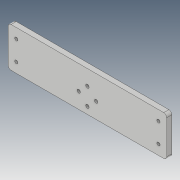
# Autodesk Inventor part: verticalAcrylicMount
Saved by Autodesk Inventor 2018 (Build 220112000, 112)
## iProperties
Created: 2020-02-23
Part Number: verticalAcrylicMount
Material: Generic
Document SubType Name: Modeling
Designer: anirudh
Density: 1 g/cm^3
Appearance: Default
Author: anirudh
Autodesk Inventor part; units mm, degrees
ref_plane "YZ Plane" through (0, 0, 0) normal (1, 0, 0) x (0, 1, 0)
ref_plane "XZ Plane" through (0, 0, 0) normal (0, 1, 0) x (-1, 0, 0)
ref_plane "XY Plane" through (0, 0, 0) normal (0, 0, 1) x (1, 0, 0)
sketch "Sketch1" plane through (0, 0, 0) normal (0, 0, 1) x (1, 0, 0)
  line L0 (0, 0) -> (149.225, 0)
  line L1 (149.225, 0) -> (149.225, -43.1292)
  line L2 (149.225, -43.1292) -> (0, -43.1292)
  line L3 (0, -43.1292) -> (0, 0)
  circle A0 centre (65.1125, -26.01) radius 1.85
  circle A1 centre (65.1125, -26.01) radius 1.85
  circle A2 centre (74.6125, -35.51) radius 1.85
  circle A3 centre (74.6125, -35.51) radius 1.85
  circle A4 centre (84.1125, -26.01) radius 1.85
  circle A5 centre (84.1125, -26.01) radius 1.85
  circle A6 centre (74.6125, -16.51) radius 1.85
  circle A7 centre (74.6125, -16.51) radius 1.85
  line L4 (0, 0) -> (8.89, 0)
  line L5 (149.225, 0) -> (140.335, 0)
  circle A8 centre (8.89, -10.7823) radius 1.75
  circle A9 centre (8.89, -32.3469) radius 1.75
  circle A10 centre (140.335, -10.7823) radius 1.75
  circle A11 centre (140.335, -32.3469) radius 1.75
  dimension "d0" = 149.225
  dimension "d1" = 43.1292
  dimension "d3" = 8.89
  dimension "d4" = 8.89
  dimension "d5" = 3.5
  dimension "d6" = 3.5
  dimension "d7" = 3.5
  dimension "d8" = 3.5
  constraints: 12 centre point, 12 end point, 4 coincident, 2 parallel, 2 point on line, 1 horizontal, 1 perpendicular
  measures "d0" distance of L1.end L2.end
  measures "d1" distance of L0.end L1.end
  measures "d3" distance of L0.start L4.end
  measures "d4" distance of L0.end L5.end
  measures "d5" diameter of A8
  measures "d6" diameter of A9
  measures "d7" diameter of A10
  measures "d8" diameter of A11
extrude "Extrusion1" add sketch "Sketch1" along normal blind 5.588
sketch "Sketch2" plane through (0, 0, 5.588) normal (0, 0, 1) x (1, 0, 0)
  line L0 (149.225, 0) -> (0, 0) projected
  line L1 (0, 0) -> (-11.4173, 0)
  line L2 (-11.4173, 0) -> (-11.4173, -43.1292)
  line L3 (-11.4173, -43.1292) -> (0, -43.1292)
  line L4 (0, -43.1292) -> (0, 0)
  line L5 (149.225, -43.1292) -> (149.225, 0) projected
  line L6 (149.225, 0) -> (160.6423, 0)
  line L7 (160.6423, 0) -> (160.6423, -43.1292)
  line L8 (160.6423, -43.1292) -> (149.225, -43.1292)
  line L9 (149.225, -43.1292) -> (149.225, 0)
  dimension "d12" = 11.4173
  dimension "d13" = 11.4173
  constraints: 16 end point, 4 parallel, 2 horizontal, 2 perpendicular
  measures "d12" distance of L3.end L2.end
  measures "d13" distance of L7.end L8.end
extrude "Extrusion2" add sketch "Sketch2" against normal blind 5.588
sketch "Sketch3" plane through (0, 0, 5.588) normal (0, 0, 1) x (1, 0, 0)
  line L0 (-11.4173, -43.1292) -> (-11.4173, 0) projected
  circle A0 centre (8.89, -10.7823) radius 1.75 projected
  circle A1 centre (8.89, -32.3469) radius 1.75 projected
  circle A2 centre (140.335, -10.7823) radius 1.75 projected
  circle A3 centre (140.335, -32.3469) radius 1.75 projected
  line L1 (160.6423, 0) -> (160.6423, -43.1292) projected
  circle A4 centre (-2.5273, -10.7823) radius 1.75
  circle A5 centre (-2.5273, -32.3469) radius 1.75
  circle A6 centre (151.7523, -10.7823) radius 1.75
  circle A7 centre (151.7523, -32.3469) radius 1.75
  point P0 (0, 0)
  constraints: 4 centre point
sketch "Sketch4" plane through (0, 0, 5.588) normal (0, 0, 1) x (1, 0, 0)
  circle A0 centre (8.89, -10.7823) radius 1.75 projected
  circle A1 centre (8.89, -10.7823) radius 5.9752
  circle A2 centre (8.89, -32.3469) radius 1.75 projected
  circle A3 centre (8.89, -32.3469) radius 5.6111
  circle A4 centre (140.335, -10.7823) radius 1.75 projected
  circle A5 centre (140.335, -10.7823) radius 4.3927
  circle A6 centre (140.335, -32.3469) radius 1.75 projected
  circle A7 centre (140.335, -32.3469) radius 4.6933
  point P0 (0, 0)
  constraints: 4 centre point, 4 coincident
extrude "Extrusion3" add sketch "Sketch4" against normal blind 5.588 contours A0 | A1 | A2 | A3 | A4 | A5 | A6 | A7
extrude "Extrusion4" cut sketch "Sketch3" against normal blind 62.6745 contours A4 | A5 | A6 | A7
fillet "Fillet2" radius 3.175 4 edges at (-11.4173, -43.1292, 2.794) (-11.4173, 0, 2.794) (160.6423, -43.1292, 2.794) (160.6423, 0, 2.794)
body "Solid1"
